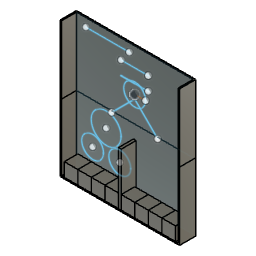
resistor bot v1 (Autodesk Fusion 360 design; units mm, degrees)
Autodesk Fusion 360 part; units mm, degrees
box "BoxPrimitive1" add length 12 width 44 height 50 placed x (0, 1, 0) y (-1, 0, 0) z (0, 0, 1) at (22, -11, 0) makes body 1
move_body "Move1" bodies 1 to x (1, 0, 0) y (0, 1, 0) z (0, 0, 1) at (0, 5, 0)
split "Split1" by plane through (0, 0, 0) normal (0, 1, 0) bodies 1 makes body 2 at (7.3333, 6, 16.6667)
move_body "Move9" bodies 1 to x (1, 0, 0) y (0, 1, 0) z (0, 0, 1) at (0, 6, 0)
shell "Shell2" thickness 0.5 removed faces 2 at (-7.3333, 2, 50) at (7.3333, 0, 16.6667) on bodies 1
box "BoxPrimitive3" add length 5 width 5 height 5 placed x (0, -1, 0) y (1, 0, 0) z (0, 0, 1) at (-21, 5, 0.5) separate body makes body 3
delete_body "RemoveBody18" bodies 2
ref_plane "WorkPlane1" through (0, 0, 25) normal (0, 0, 1) x (1, 0, 0)
box "BoxPrimitive4" add length 5.5 width 1 height 39.5 placed x (0, 1, 0) y (-1, 0, 0) z (0, 0, 1) at (0.5, 0, 0.5) separate body makes body 4
split "Split2" by plane through (0, 0, 25) normal (0, 0, 1) bodies 1 4 makes body 6 at (0.5, 3.6667, 30) makes body 5 at (7.3333, 6, 33.3333)
move_body "Move10" bodies 3 to x (1, 0, 0) y (0, 1, 0) z (0, 0, 1) at (0.5, 0, 0)
sketch "Sketch8" plane through (0, 5.5, 0) normal (0, -1, 0) x (1, 0, 0)
  line L0 (21.5, 25) -> (-21.5, 25)
  line L1 (-21.5, 25) -> (-21.5, 0.5)
  line L2 (-21.5, 0.5) -> (21.5, 0.5)
  line L3 (21.5, 0.5) -> (21.5, 25)
  circle A0 centre (-15.5, 10) radius 4
  circle A1 centre (-5.5, 10) radius 4
  circle A2 centre (-10.5, 18.5) radius 5.5
copy_body "CopyPasteBodies5" bodies 3 makes body 7
move_body "Move11" bodies 7 to x (1, 0, 0) y (0, 1, 0) z (0, 0, 1) at (5, 0, 0)
copy_body "CopyPasteBodies6" bodies 7 3 makes body 8 makes body 9
move_body "Move12" bodies 8 9 to x (1, 0, 0) y (0, 1, 0) z (0, 0, 1) at (10, 0, 0)
copy_body "CopyPasteBodies7" bodies 3 7 9 8 makes body 10 makes body 11 makes body 12 makes body 13
move_body "Move13" bodies 10 11 12 13 to x (1, 0, 0) y (0, 1, 0) z (0, 0, 1) at (21, 0, 0)
delete_body "RemoveBody19" bodies 6
move_face "OffsetFaces1" offset -5 1 faces at (-0.1667, 3.6667, 25) on bodies 4
sketch "Sketch12" plane through (0, 5.5, 0) normal (0, -1, 0) x (1, 0, 0)
  line L0 (-21.5, 25) -> (21.5, 25)
  line L1 (21.5, 25) -> (21.5, 50)
  line L2 (21.5, 50) -> (-21.5, 50)
  line L3 (-21.5, 50) -> (-21.5, 25)
  line L4 (0, 33) -> (-8.4853, 24.5147)
  line L5 (0, 33) -> (8.4853, 24.5147)
  circle A0 centre (0, 34.5) radius 4
  line L6 (0, 34.5) -> (4, 34.5) construction
  line L7 (5, 38) -> (-5, 38)
  line L8 (-5, 38) -> (0, 38)
  line L9 (-5, 43) -> (5, 43)
  line L10 (-18, 47) -> (-2, 47)
  dimension "d61" = 12
  constraint perpendicular L4 L5
  constraint horizontal L6
  constraint coincident A0.centre L6.start
  constraint horizontal L7
  constraint midpoint L7 L8.end
  constraint horizontal L9
  constraint horizontal L10
  measures "d61" distance of L4.start L5.end
sketch "Sketch13" plane through (0, 5.5, 0) normal (0, -1, 0) x (1, 0, 0)
named bodies: "lower part", "frame (1)", "example box", "upper part", "example box (1)", "example box (2)", "example box (1) (1)", "example box (3)", "example box (2) (1)", "example box (1) (1) (1)", "example box (1) (1) (1) (1)"
